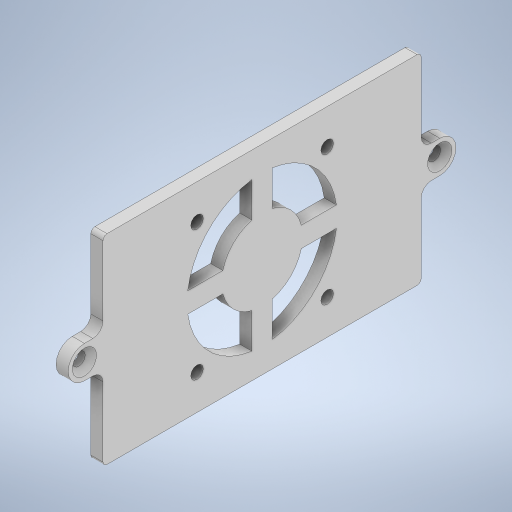
# Autodesk Inventor part: pokrywa_przod
Saved by Autodesk Inventor 2023.4 (Build 274418000, 418)
## iProperties
Created: 2024-07-28
Part Number: pokrywa_przod
Material: Ogólny
Document SubType Name: Modeling
Designer: kamil
Density: 1 g/cm^3
Appearance: Domyślna
Author: kamil
Autodesk Inventor part; units mm, degrees
ref_plane "YZ Plane" through (0, 0, 0) normal (1, 0, 0) x (0, 1, 0)
ref_plane "XZ Plane" through (0, 0, 0) normal (0, 1, 0) x (-1, 0, 0)
ref_plane "XY Plane" through (0, 0, 0) normal (0, 0, 1) x (1, 0, 0)
sketch "Szkic1" plane through (0, 0, 0) normal (1, 0, 0) x (0, 1, 0)
  line L0 (6.2889, -7.1741) -> (-43.0111, -7.1741)
  line L1 (-43.0111, -7.1741) -> (-43.0111, -85.6741)
  line L2 (-43.0111, -85.6741) -> (6.2889, -85.6741)
  line L3 (6.2889, -85.6741) -> (6.2889, -7.1741)
  point P0 (0, 0)
  dimension "d0" = 49.3
  dimension "d1" = 78.5
  constraints: 8 end point, 2 parallel, 1 horizontal, 1 perpendicular
  measures "d0" distance of L2.end L1.end
  measures "d1" distance of L1.end L0.end
extrude "Wyciągnięcie proste1" add sketch "Szkic1" along normal blind 3
sketch "Sketch3" plane through (3, 0, 0) normal (1, 0, 0) x (0, 0, -1)
  arc A0 (2.5987, -14.1111) -> (2.5987, -22.6111) centre (2.5987, -18.3611) ccw
  arc A1 (90.2495, -22.6111) -> (90.2495, -14.1111) centre (90.2495, -18.3611) ccw
  line L0 (90.2495, -14.1111) -> (88.4995, -14.1111)
  line L1 (90.2495, -22.6111) -> (88.4995, -22.6111)
  line L2 (2.5987, -14.1111) -> (4.3487, -14.1111)
  line L3 (4.3487, -22.6111) -> (2.5987, -22.6111)
  line L4 (7.1741, -43.0111) -> (85.6741, -43.0111)
  line L5 (85.6741, -43.0111) -> (85.6741, 6.2889)
  line L6 (85.6741, 6.2889) -> (7.1741, 6.2889)
  line L7 (7.1741, 6.2889) -> (7.1741, -43.0111)
  line L8 (4.3487, -22.6111) -> (7.1741, -22.6111)
  line L9 (7.1741, 6.2889) -> (7.1741, -43.0111)
  line L10 (4.3487, -14.1111) -> (7.1741, -14.1111)
  line L11 (88.4995, -14.1111) -> (85.6741, -14.1111)
  line L12 (88.4995, -22.6111) -> (85.6741, -22.6111)
  line L13 (85.6741, -14.3611) -> (88.4995, -14.3611)
  line L14 (88.4995, -14.3611) -> (90.2495, -14.3611)
  arc A2 (90.2495, -22.3611) -> (90.2495, -14.3611) centre (90.2495, -18.3611) ccw
  line L15 (90.2495, -22.3611) -> (88.4995, -22.3611)
  line L16 (88.4995, -22.3611) -> (85.6741, -22.3611)
  line L17 (7.1741, -22.3611) -> (4.3487, -22.3611)
  line L18 (4.3487, -22.3611) -> (2.5987, -22.3611)
  arc A3 (2.5987, -14.3611) -> (2.5987, -22.3611) centre (2.5987, -18.3611) ccw
  line L19 (2.5987, -14.3611) -> (4.3487, -14.3611)
  line L20 (4.3487, -14.3611) -> (7.1741, -14.3611)
  point P0 (0, 0)
extrude "Extrusion2" add sketch "Sketch3" against normal blind 3 contours L7 L17 L18 A3 L19 L20 | L13 L14 A2 L15 L16 L5
sketch "Sketch4" plane through (3, 0, 0) normal (1, 0, 0) x (0, 0, -1)
  arc A0 (2.5987, -14.3611) -> (2.5987, -22.3611) centre (2.5987, -18.3611) ccw projected
  arc A1 (90.2495, -22.3611) -> (90.2495, -14.3611) centre (90.2495, -18.3611) ccw projected
  point P0 (0, 0)
hole "Hole2" at (3, -18.3611, -90.2495) at (3, -18.3611, -2.5987) direction (-1, 0, 0) diameter 3.2 end through all countersink diameter 6 countersink angle 90
fillet "Fillet2" radius 2.5 4 edges at (1.5, -22.3611, -85.6741) (1.5, -14.3611, -85.6741) (1.5, -22.3611, -7.1741) (1.5, -14.3611, -7.1741)
fillet "Fillet3" radius 1 4 edges at (1.5, -43.0111, -85.6741) (1.5, -43.0111, -7.1741) (1.5, 6.2889, -85.6741) (1.5, 6.2889, -7.1741)
sketch "Sketch5" plane through (0, 0, 0) normal (-1, 0, 0) x (0, 0, 1)
  circle A0 centre (-90.2495, -18.3611) radius 1.6 projected
  circle A1 centre (-2.5987, -18.3611) radius 1.6 projected
  arc A2 (-7.1741, 5.2889) -> (-8.1741, 6.2889) centre (-8.1741, 5.2889) ccw projected
  line L0 (-84.6741, 6.2889) -> (-8.1741, 6.2889) projected
  arc A3 (-84.6741, 6.2889) -> (-85.6741, 5.2889) centre (-84.6741, 5.2889) ccw projected
  line L1 (-85.6741, -11.8611) -> (-85.6741, 5.2889) projected
  arc A4 (-88.1741, -14.3611) -> (-85.6741, -11.8611) centre (-88.1741, -11.8611) ccw projected
  line L2 (-88.1741, -14.3611) -> (-90.2495, -14.3611) projected
  arc A5 (-90.2495, -14.3611) -> (-90.2495, -22.3611) centre (-90.2495, -18.3611) ccw projected
  line L3 (-90.2495, -22.3611) -> (-88.1741, -22.3611) projected
  arc A6 (-85.6741, -24.8611) -> (-88.1741, -22.3611) centre (-88.1741, -24.8611) ccw projected
  line L4 (-85.6741, -42.0111) -> (-85.6741, -24.8611) projected
  arc A7 (-85.6741, -42.0111) -> (-84.6741, -43.0111) centre (-84.6741, -42.0111) ccw projected
  line L5 (-8.1741, -43.0111) -> (-84.6741, -43.0111) projected
  arc A8 (-8.1741, -43.0111) -> (-7.1741, -42.0111) centre (-8.1741, -42.0111) ccw projected
  line L6 (-7.1741, -24.8611) -> (-7.1741, -42.0111) projected
  arc A9 (-4.6741, -22.3611) -> (-7.1741, -24.8611) centre (-4.6741, -24.8611) ccw projected
  line L7 (-4.6741, -22.3611) -> (-2.5987, -22.3611) projected
  arc A10 (-2.5987, -22.3611) -> (-2.5987, -14.3611) centre (-2.5987, -18.3611) ccw projected
  line L8 (-2.5987, -14.3611) -> (-4.6741, -14.3611) projected
  arc A11 (-7.1741, -11.8611) -> (-4.6741, -14.3611) centre (-4.6741, -11.8611) ccw projected
  line L9 (-7.1741, 5.2889) -> (-7.1741, -11.8611) projected
  line L10 (-26.4241, -38.3611) -> (-66.4241, -38.3611)
  line L11 (-66.4241, -38.3611) -> (-66.4241, 1.6389)
  line L12 (-66.4241, 1.6389) -> (-26.4241, 1.6389)
  line L13 (-26.4241, 1.6389) -> (-26.4241, -38.3611)
  line L14 (-26.4241, -38.3611) -> (-66.4241, 1.6389) construction
  line L15 (-66.4241, -38.3611) -> (-26.4241, 1.6389) construction
  line L16 (-30.3707, -34.4146) -> (-62.4776, -2.3077)
  line L17 (-62.4776, -34.4146) -> (-30.3707, -2.3077)
  point P0 (0, 0)
  point P1 (-46.4241, 6.2889)
  point P2 (-46.4241, -18.3611)
  dimension "d26" = 40
  dimension "d27" = 40
  dimension "d28" = 45.406
  dimension "d29" = 45.406
  constraints: 16 end point, 5 midpoint, 2 coincident, 2 parallel, 2 perpendicular, 2 point on line, 1 collinear, 1 horizontal, 1 horizontal alignment, 1 vertical alignment
  measures "d26" distance of L11.end L12.end
  measures "d27" distance of L10.end L11.end
  measures "d28" distance of L16.start L16.end
  measures "d29" distance of L17.end L17.start
hole "Hole3" at (0, -34.4146, -62.4776) at (0, -2.3077, -62.4776) at (0, -34.4146, -30.3707) at (0, -2.3077, -30.3707) direction (1, 0, 0) diameter 3.1 end through all
sketch "Sketch6" plane through (0, 0, 0) normal (-1, 0, 0) x (0, 0, 1)
  circle A0 centre (-30.3707, -34.4146) radius 1.55 projected
  circle A1 centre (-62.4776, -34.4146) radius 1.55 projected
  circle A2 centre (-62.4776, -2.3077) radius 1.55 projected
  circle A3 centre (-30.3707, -2.3077) radius 1.55 projected
  circle A4 centre (-90.2495, -18.3611) radius 1.6 projected
  circle A5 centre (-2.5987, -18.3611) radius 1.6 projected
  arc A6 (-7.1741, 5.2889) -> (-8.1741, 6.2889) centre (-8.1741, 5.2889) ccw projected
  line L0 (-84.6741, 6.2889) -> (-8.1741, 6.2889) projected
  arc A7 (-84.6741, 6.2889) -> (-85.6741, 5.2889) centre (-84.6741, 5.2889) ccw projected
  line L1 (-85.6741, -11.8611) -> (-85.6741, 5.2889) projected
  arc A8 (-88.1741, -14.3611) -> (-85.6741, -11.8611) centre (-88.1741, -11.8611) ccw projected
  line L2 (-88.1741, -14.3611) -> (-90.2495, -14.3611) projected
  arc A9 (-90.2495, -14.3611) -> (-90.2495, -22.3611) centre (-90.2495, -18.3611) ccw projected
  line L3 (-90.2495, -22.3611) -> (-88.1741, -22.3611) projected
  arc A10 (-85.6741, -24.8611) -> (-88.1741, -22.3611) centre (-88.1741, -24.8611) ccw projected
  line L4 (-85.6741, -42.0111) -> (-85.6741, -24.8611) projected
  arc A11 (-85.6741, -42.0111) -> (-84.6741, -43.0111) centre (-84.6741, -42.0111) ccw projected
  line L5 (-8.1741, -43.0111) -> (-84.6741, -43.0111) projected
  arc A12 (-8.1741, -43.0111) -> (-7.1741, -42.0111) centre (-8.1741, -42.0111) ccw projected
  line L6 (-7.1741, -24.8611) -> (-7.1741, -42.0111) projected
  arc A13 (-4.6741, -22.3611) -> (-7.1741, -24.8611) centre (-4.6741, -24.8611) ccw projected
  line L7 (-4.6741, -22.3611) -> (-2.5987, -22.3611) projected
  arc A14 (-2.5987, -22.3611) -> (-2.5987, -14.3611) centre (-2.5987, -18.3611) ccw projected
  line L8 (-2.5987, -14.3611) -> (-4.6741, -14.3611) projected
  arc A15 (-7.1741, -11.8611) -> (-4.6741, -14.3611) centre (-4.6741, -11.8611) ccw projected
  line L9 (-7.1741, 5.2889) -> (-7.1741, -11.8611) projected
  circle A16 centre (-62.4776, -2.3077) radius 1.55 projected
  circle A17 centre (-30.3707, -34.4146) radius 1.55 projected
  line L10 (-62.4776, -2.3077) -> (-30.3707, -34.4146)
  circle A18 centre (-62.4776, -34.4146) radius 1.55 projected
  circle A19 centre (-46.4241, -18.3611) radius 19.5
  circle A20 centre (-46.4241, -18.3611) radius 18.5
  point P0 (0, 0)
  point P1 (-46.4241, -18.3611)
  dimension "d37" = 39
  dimension "d38" = 1
  constraints: 2 centre point, 2 coincident, 2 end point, 1 midpoint
  measures "d37" diameter of A19
  measures "d38" radial gap between concentric circles of A19 A20
extrude "Extrusion3" cut sketch "Sketch6" against normal through all contours A20 L10 | L10 A20
sketch "Sketch7" plane through (0, 0, 0) normal (-1, 0, 0) x (0, 0, 1)
  circle A0 centre (-46.4241, -18.3611) radius 18.5 projected
  circle A1 centre (-46.4241, -18.3611) radius 10
  line L0 (-64.9241, -15.8611) -> (-27.9241, -15.8611)
  line L1 (-27.9241, -15.8611) -> (-27.9241, -20.8611)
  line L2 (-27.9241, -20.8611) -> (-64.9241, -20.8611)
  line L3 (-64.9241, -20.8611) -> (-64.9241, -15.8611)
  line L4 (-64.9241, -15.8611) -> (-27.9241, -20.8611) construction
  line L5 (-27.9241, -15.8611) -> (-64.9241, -20.8611) construction
  line L6 (-43.9241, -36.8611) -> (-48.9241, -36.8611)
  line L7 (-48.9241, -36.8611) -> (-48.9241, 0.1389)
  line L8 (-48.9241, 0.1389) -> (-43.9241, 0.1389)
  line L9 (-43.9241, 0.1389) -> (-43.9241, -36.8611)
  line L10 (-43.9241, -36.8611) -> (-48.9241, 0.1389) construction
  line L11 (-48.9241, -36.8611) -> (-43.9241, 0.1389) construction
  point P0 (0, 0)
  point P1 (-43.9241, -8.6787)
  point P2 (-43.9241, -0.0308)
  point P3 (-48.9241, -0.0308)
  point P4 (-48.9241, -8.6787)
  point P5 (-56.1066, -15.8611)
  point P6 (-64.7544, -15.8611)
  point P7 (-64.7544, -20.8611)
  point P8 (-56.1066, -20.8611)
  point P9 (-48.9241, -28.0436)
  point P10 (-48.9241, -36.6914)
  point P11 (-43.9241, -36.6914)
  point P12 (-43.9241, -28.0436)
  point P13 (-36.7416, -20.8611)
  point P14 (-28.0938, -20.8611)
  point P15 (-28.0938, -15.8611)
  point P16 (-36.7416, -15.8611)
  dimension "d41" = 20
  dimension "d42" = 5
  dimension "d43" = 5
  constraints: 24 end point, 4 midpoint, 4 parallel, 2 horizontal, 2 perpendicular, 2 tangent, 1 centre point, 1 coincident
  measures "d41" diameter of A1
  measures "d42" distance of L0.end L1.end
  measures "d43" distance of L7.end L8.end
extrude "Extrusion4" add sketch "Sketch7" against normal up to surface (3 mm away) contours A0 L2 A1 L0 | L9 A1 L7 A0 | L0 L9 A1 | A1 L2 L9 L0 | A0 L7 A1 L9 | A1 L9 L2 | L9 L0 L7 A1 | L9 L2 L7 L0 | A1 L7 L2 L9 | L7 L0 A1 | L7 L2 A1 L0 | A1 L2 L7 | L0 A1 L2 A0
